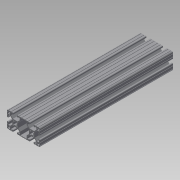
# Autodesk Inventor part: 1530-UL
Saved by Autodesk Inventor 2013 (Build 170138000, 138)
## iProperties
Company: 80/20 Inc.
Created: 2014-04-23
Part Number: 1530-UL
Material: Generic
Document SubType Name: Modeling
Density: 1 g/cm^3
Vendor: 80/20 Inc.
Engineer: Ross Bowman
Designer: Ross Bowman
Catalog Web Link: 8020.net
Material: 6105-T5 Aluminum
Author: Ross Bowman
Keywords: 80/20 , 8020 , T-Slot , Extrusion
Autodesk Inventor part; units mm, degrees
ref_plane "YZ Plane" through (0, 0, 0) normal (1, 0, 0) x (0, 1, 0)
ref_plane "XZ Plane" through (0, 0, 0) normal (0, 1, 0) x (-1, 0, 0)
ref_plane "XY Plane" through (0, 0, 0) normal (0, 0, 1) x (1, 0, 0)
sketch "Sketch1" plane through (0, 0, 0) normal (0, 0, 1) x (1, 0, 0)
  arc A0 (17.2466, -12.2428) -> (16.8656, -11.8618) centre (16.8656, -12.2428) ccw
  line L0 (17.2466, -14.4526) -> (17.2466, -12.2428)
  arc A1 (14.4526, -17.2466) -> (17.2466, -14.4526) centre (14.4526, -14.4526) ccw
  line L1 (12.2428, -17.2466) -> (14.4526, -17.2466)
  arc A2 (11.8618, -16.8656) -> (12.2428, -17.2466) centre (12.2428, -16.8656) ccw
  line L2 (11.8618, -15.0876) -> (11.8618, -16.8656)
  line L3 (12.3952, -14.5542) -> (11.8618, -15.0876)
  line L4 (11.8618, -14.0208) -> (12.3952, -14.5542)
  line L5 (11.8618, -12.2428) -> (11.8618, -14.0208)
  arc A3 (12.2428, -11.8618) -> (11.8618, -12.2428) centre (12.2428, -12.2428) ccw
  line L6 (14.0208, -11.8618) -> (12.2428, -11.8618)
  line L7 (14.5542, -12.3952) -> (14.0208, -11.8618)
  line L8 (15.0876, -11.8618) -> (14.5542, -12.3952)
  line L9 (16.8656, -11.8618) -> (15.0876, -11.8618)
  arc A4 (-3.1119, 1.178) -> (-3.1119, -1.178) centre (0, 0) ccw
  arc A5 (-3.1119, 1.178) -> (-3.1988, 1.5823) centre (-3.4682, 1.3129) ccw
  line L10 (-4.9085, 3.2921) -> (-3.1988, 1.5823)
  arc A6 (-5.1689, 3.9207) -> (-4.9085, 3.2921) centre (-4.2799, 3.9207) ccw
  line L11 (-5.1689, 4.9149) -> (-5.1689, 3.9207)
  arc A7 (-4.9149, 5.1689) -> (-5.1689, 4.9149) centre (-4.9149, 4.9149) ccw
  line L12 (-3.9207, 5.1689) -> (-4.9149, 5.1689)
  arc A8 (-3.2921, 4.9085) -> (-3.9207, 5.1689) centre (-3.9207, 4.2799) ccw
  line L13 (-1.5823, 3.1988) -> (-3.2921, 4.9085)
  arc A9 (-1.5823, 3.1988) -> (-1.178, 3.1119) centre (-1.3129, 3.4682) ccw
  arc A10 (1.178, 3.1119) -> (-1.178, 3.1119) centre (0, 0) ccw
  arc A11 (1.178, 3.1119) -> (1.5823, 3.1988) centre (1.3129, 3.4682) ccw
  line L14 (3.2921, 4.9085) -> (1.5823, 3.1988)
  arc A12 (3.9207, 5.1689) -> (3.2921, 4.9085) centre (3.9207, 4.2799) ccw
  line L15 (4.9149, 5.1689) -> (3.9207, 5.1689)
  arc A13 (5.1689, 4.9149) -> (4.9149, 5.1689) centre (4.9149, 4.9149) ccw
  line L16 (5.1689, 3.9207) -> (5.1689, 4.9149)
  arc A14 (4.9085, 3.2921) -> (5.1689, 3.9207) centre (4.2799, 3.9207) ccw
  line L17 (3.1988, 1.5823) -> (4.9085, 3.2921)
  arc A15 (3.1988, 1.5823) -> (3.1119, 1.178) centre (3.4682, 1.3129) ccw
  arc A16 (3.1119, -1.178) -> (3.1119, 1.178) centre (0, 0) ccw
  arc A17 (3.1119, -1.178) -> (3.1988, -1.5823) centre (3.4682, -1.3129) ccw
  line L18 (4.9085, -3.2921) -> (3.1988, -1.5823)
  arc A18 (5.1689, -3.9207) -> (4.9085, -3.2921) centre (4.2799, -3.9207) ccw
  line L19 (5.1689, -4.9149) -> (5.1689, -3.9207)
  arc A19 (4.9149, -5.1689) -> (5.1689, -4.9149) centre (4.9149, -4.9149) ccw
  line L20 (3.9207, -5.1689) -> (4.9149, -5.1689)
  arc A20 (3.2921, -4.9085) -> (3.9207, -5.1689) centre (3.9207, -4.2799) ccw
  line L21 (1.5823, -3.1988) -> (3.2921, -4.9085)
  arc A21 (1.5823, -3.1988) -> (1.178, -3.1119) centre (1.3129, -3.4682) ccw
  arc A22 (-1.178, -3.1119) -> (1.178, -3.1119) centre (0, 0) ccw
  arc A23 (-1.178, -3.1119) -> (-1.5823, -3.1988) centre (-1.3129, -3.4682) ccw
  line L22 (-3.2921, -4.9085) -> (-1.5823, -3.1988)
  arc A24 (-3.9207, -5.1689) -> (-3.2921, -4.9085) centre (-3.9207, -4.2799) ccw
  line L23 (-4.9149, -5.1689) -> (-3.9207, -5.1689)
  arc A25 (-5.1689, -4.9149) -> (-4.9149, -5.1689) centre (-4.9149, -4.9149) ccw
  line L24 (-5.1689, -3.9207) -> (-5.1689, -4.9149)
  arc A26 (-4.9085, -3.2921) -> (-5.1689, -3.9207) centre (-4.2799, -3.9207) ccw
  line L25 (-3.1988, -1.5823) -> (-4.9085, -3.2921)
  arc A27 (-3.1988, -1.5823) -> (-3.1119, -1.178) centre (-3.4682, -1.3129) ccw
  arc A28 (-41.2119, 1.178) -> (-41.2119, -1.178) centre (-38.1, 0) ccw
  arc A29 (-41.2119, 1.178) -> (-41.2988, 1.5823) centre (-41.5682, 1.3129) ccw
  line L26 (-43.0085, 3.2921) -> (-41.2988, 1.5823)
  arc A30 (-43.2689, 3.9207) -> (-43.0085, 3.2921) centre (-42.3799, 3.9207) ccw
  line L27 (-43.2689, 4.9149) -> (-43.2689, 3.9207)
  arc A31 (-43.0149, 5.1689) -> (-43.2689, 4.9149) centre (-43.0149, 4.9149) ccw
  line L28 (-42.0207, 5.1689) -> (-43.0149, 5.1689)
  arc A32 (-41.3921, 4.9085) -> (-42.0207, 5.1689) centre (-42.0207, 4.2799) ccw
  line L29 (-39.6823, 3.1988) -> (-41.3921, 4.9085)
  arc A33 (-39.6823, 3.1988) -> (-39.278, 3.1119) centre (-39.4129, 3.4682) ccw
  arc A34 (-36.922, 3.1119) -> (-39.278, 3.1119) centre (-38.1, 0) ccw
  arc A35 (-36.922, 3.1119) -> (-36.5177, 3.1988) centre (-36.7871, 3.4682) ccw
  line L30 (-34.8079, 4.9085) -> (-36.5177, 3.1988)
  arc A36 (-34.1793, 5.1689) -> (-34.8079, 4.9085) centre (-34.1793, 4.2799) ccw
  line L31 (-33.1851, 5.1689) -> (-34.1793, 5.1689)
  arc A37 (-32.9311, 4.9149) -> (-33.1851, 5.1689) centre (-33.1851, 4.9149) ccw
  line L32 (-32.9311, 3.9207) -> (-32.9311, 4.9149)
  arc A38 (-33.1915, 3.2921) -> (-32.9311, 3.9207) centre (-33.8201, 3.9207) ccw
  line L33 (-34.9012, 1.5823) -> (-33.1915, 3.2921)
  arc A39 (-34.9012, 1.5823) -> (-34.9881, 1.178) centre (-34.6318, 1.3129) ccw
  arc A40 (-34.9881, -1.178) -> (-34.9881, 1.178) centre (-38.1, 0) ccw
  arc A41 (-34.9881, -1.178) -> (-34.9012, -1.5823) centre (-34.6318, -1.3129) ccw
  line L34 (-33.1915, -3.2921) -> (-34.9012, -1.5823)
  arc A42 (-32.9311, -3.9207) -> (-33.1915, -3.2921) centre (-33.8201, -3.9207) ccw
  line L35 (-32.9311, -4.9149) -> (-32.9311, -3.9207)
  arc A43 (-33.1851, -5.1689) -> (-32.9311, -4.9149) centre (-33.1851, -4.9149) ccw
  line L36 (-34.1793, -5.1689) -> (-33.1851, -5.1689)
  arc A44 (-34.8079, -4.9085) -> (-34.1793, -5.1689) centre (-34.1793, -4.2799) ccw
  line L37 (-36.5177, -3.1988) -> (-34.8079, -4.9085)
  arc A45 (-36.5177, -3.1988) -> (-36.922, -3.1119) centre (-36.7871, -3.4682) ccw
  arc A46 (-39.278, -3.1119) -> (-36.922, -3.1119) centre (-38.1, 0) ccw
  arc A47 (-39.278, -3.1119) -> (-39.6823, -3.1988) centre (-39.4129, -3.4682) ccw
  line L38 (-41.3921, -4.9085) -> (-39.6823, -3.1988)
  arc A48 (-42.0207, -5.1689) -> (-41.3921, -4.9085) centre (-42.0207, -4.2799) ccw
  line L39 (-43.0149, -5.1689) -> (-42.0207, -5.1689)
  arc A49 (-43.2689, -4.9149) -> (-43.0149, -5.1689) centre (-43.0149, -4.9149) ccw
  line L40 (-43.2689, -3.9207) -> (-43.2689, -4.9149)
  arc A50 (-43.0085, -3.2921) -> (-43.2689, -3.9207) centre (-42.3799, -3.9207) ccw
  line L41 (-41.2988, -1.5823) -> (-43.0085, -3.2921)
  arc A51 (-41.2988, -1.5823) -> (-41.2119, -1.178) centre (-41.5682, -1.3129) ccw
  arc A52 (-54.9656, -11.8618) -> (-55.3466, -12.2428) centre (-54.9656, -12.2428) ccw
  line L42 (-53.1876, -11.8618) -> (-54.9656, -11.8618)
  line L43 (-52.6542, -12.3952) -> (-53.1876, -11.8618)
  line L44 (-52.1208, -11.8618) -> (-52.6542, -12.3952)
  line L45 (-50.3428, -11.8618) -> (-52.1208, -11.8618)
  arc A53 (-49.9618, -12.2428) -> (-50.3428, -11.8618) centre (-50.3428, -12.2428) ccw
  line L46 (-49.9618, -14.0208) -> (-49.9618, -12.2428)
  line L47 (-50.4952, -14.5542) -> (-49.9618, -14.0208)
  line L48 (-49.9618, -15.0876) -> (-50.4952, -14.5542)
  line L49 (-49.9618, -16.8656) -> (-49.9618, -15.0876)
  arc A54 (-50.3428, -17.2466) -> (-49.9618, -16.8656) centre (-50.3428, -16.8656) ccw
  line L50 (-52.5526, -17.2466) -> (-50.3428, -17.2466)
  arc A55 (-55.3466, -14.4526) -> (-52.5526, -17.2466) centre (-52.5526, -14.4526) ccw
  line L51 (-55.3466, -12.2428) -> (-55.3466, -14.4526)
  arc A56 (-55.3466, 12.2428) -> (-54.9656, 11.8618) centre (-54.9656, 12.2428) ccw
  line L52 (-55.3466, 14.4526) -> (-55.3466, 12.2428)
  arc A57 (-52.5526, 17.2466) -> (-55.3466, 14.4526) centre (-52.5526, 14.4526) ccw
  line L53 (-50.3428, 17.2466) -> (-52.5526, 17.2466)
  arc A58 (-49.9618, 16.8656) -> (-50.3428, 17.2466) centre (-50.3428, 16.8656) ccw
  line L54 (-49.9618, 15.0876) -> (-49.9618, 16.8656)
  line L55 (-50.4952, 14.5542) -> (-49.9618, 15.0876)
  line L56 (-49.9618, 14.0208) -> (-50.4952, 14.5542)
  line L57 (-49.9618, 12.2428) -> (-49.9618, 14.0208)
  arc A59 (-50.3428, 11.8618) -> (-49.9618, 12.2428) centre (-50.3428, 12.2428) ccw
  line L58 (-52.1208, 11.8618) -> (-50.3428, 11.8618)
  line L59 (-52.6542, 12.3952) -> (-52.1208, 11.8618)
  line L60 (-53.1876, 11.8618) -> (-52.6542, 12.3952)
  line L61 (-54.9656, 11.8618) -> (-53.1876, 11.8618)
  arc A60 (-25.8572, 17.2466) -> (-26.2382, 16.8656) centre (-25.8572, 16.8656) ccw
  line L62 (-12.2428, 17.2466) -> (-25.8572, 17.2466)
  arc A61 (-11.8618, 16.8656) -> (-12.2428, 17.2466) centre (-12.2428, 16.8656) ccw
  line L63 (-11.8618, 10.8253) -> (-11.8618, 16.8656)
  arc A62 (-11.8618, 10.8253) -> (-11.4898, 9.9273) centre (-10.5918, 10.8253) ccw
  line L64 (-7.1157, 5.5531) -> (-11.4898, 9.9273)
  arc A63 (-6.7437, 4.6551) -> (-7.1157, 5.5531) centre (-8.0137, 4.6551) ccw
  line L65 (-6.7437, -4.6551) -> (-6.7437, 4.6551)
  arc A64 (-7.1157, -5.5531) -> (-6.7437, -4.6551) centre (-8.0137, -4.6551) ccw
  line L66 (-11.4898, -9.9273) -> (-7.1157, -5.5531)
  arc A65 (-11.4898, -9.9273) -> (-11.8618, -10.8253) centre (-10.5918, -10.8253) ccw
  line L67 (-11.8618, -16.8656) -> (-11.8618, -10.8253)
  arc A66 (-12.2428, -17.2466) -> (-11.8618, -16.8656) centre (-12.2428, -16.8656) ccw
  line L68 (-25.8572, -17.2466) -> (-12.2428, -17.2466)
  arc A67 (-26.2382, -16.8656) -> (-25.8572, -17.2466) centre (-25.8572, -16.8656) ccw
  line L69 (-26.2382, -10.8253) -> (-26.2382, -16.8656)
  arc A68 (-26.2382, -10.8253) -> (-26.6102, -9.9273) centre (-27.5082, -10.8253) ccw
  line L70 (-30.9843, -5.5531) -> (-26.6102, -9.9273)
  arc A69 (-31.3563, -4.6551) -> (-30.9843, -5.5531) centre (-30.0863, -4.6551) ccw
  line L71 (-31.3563, 4.6551) -> (-31.3563, -4.6551)
  arc A70 (-30.9843, 5.5531) -> (-31.3563, 4.6551) centre (-30.0863, 4.6551) ccw
  line L72 (-26.6102, 9.9273) -> (-30.9843, 5.5531)
  arc A71 (-26.6102, 9.9273) -> (-26.2382, 10.8253) centre (-27.5082, 10.8253) ccw
  line L73 (-26.2382, 16.8656) -> (-26.2382, 10.8253)
  arc A72 (16.8656, 11.8618) -> (17.2466, 12.2428) centre (16.8656, 12.2428) ccw
  line L74 (15.0876, 11.8618) -> (16.8656, 11.8618)
  line L75 (14.5542, 12.3952) -> (15.0876, 11.8618)
  line L76 (14.0208, 11.8618) -> (14.5542, 12.3952)
  line L77 (12.2428, 11.8618) -> (14.0208, 11.8618)
  arc A73 (11.8618, 12.2428) -> (12.2428, 11.8618) centre (12.2428, 12.2428) ccw
  line L78 (11.8618, 14.0208) -> (11.8618, 12.2428)
  line L79 (12.3952, 14.5542) -> (11.8618, 14.0208)
  line L80 (11.8618, 15.0876) -> (12.3952, 14.5542)
  line L81 (11.8618, 16.8656) -> (11.8618, 15.0876)
  arc A74 (12.2428, 17.2466) -> (11.8618, 16.8656) centre (12.2428, 16.8656) ccw
  line L82 (14.4526, 17.2466) -> (12.2428, 17.2466)
  arc A75 (17.2466, 14.4526) -> (14.4526, 17.2466) centre (14.4526, 14.4526) ccw
  line L83 (17.2466, 12.2428) -> (17.2466, 14.4526)
  arc A76 (-15.8496, 19.05) -> (-14.3256, 19.05) centre (-15.0876, 19.05) ccw
  line L84 (-15.8496, 19.05) -> (-22.2504, 19.05)
  arc A77 (-23.7744, 19.05) -> (-22.2504, 19.05) centre (-23.0124, 19.05) ccw
  line L85 (-23.7744, 19.05) -> (-28.6004, 19.05)
  arc A78 (-30.1244, 19.05) -> (-28.6004, 19.05) centre (-29.3624, 19.05) ccw
  line L86 (-30.1244, 19.05) -> (-32.4612, 19.05)
  arc A79 (-32.4612, 19.05) -> (-34.036, 17.4752) centre (-32.4612, 17.4752) ccw
  line L87 (-34.036, 17.4752) -> (-34.036, 16.5608)
  arc A80 (-34.036, 16.5608) -> (-32.4612, 14.986) centre (-32.4612, 16.5608) ccw
  line L88 (-32.4612, 14.986) -> (-31.623, 14.986)
  arc A81 (-31.623, 14.986) -> (-31.242, 15.367) centre (-31.623, 15.367) ccw
  line L89 (-31.242, 15.367) -> (-31.242, 15.6972)
  arc A82 (-30.861, 16.0782) -> (-31.242, 15.6972) centre (-30.861, 15.6972) ccw
  line L90 (-30.861, 16.0782) -> (-28.702, 16.0782)
  arc A83 (-27.813, 15.1892) -> (-28.702, 16.0782) centre (-28.702, 15.1892) ccw
  line L91 (-27.813, 15.1892) -> (-27.813, 12.3756)
  arc A84 (-28.185, 11.4776) -> (-27.813, 12.3756) centre (-29.083, 12.3756) ccw
  line L92 (-28.185, 11.4776) -> (-32.5469, 7.1157)
  arc A85 (-33.4449, 6.7437) -> (-32.5469, 7.1157) centre (-33.4449, 8.0137) ccw
  line L93 (-33.4449, 6.7437) -> (-42.7551, 6.7437)
  arc A86 (-43.6531, 7.1157) -> (-42.7551, 6.7437) centre (-42.7551, 8.0137) ccw
  line L94 (-43.6531, 7.1157) -> (-48.015, 11.4776)
  arc A87 (-48.387, 12.3756) -> (-48.015, 11.4776) centre (-47.117, 12.3756) ccw
  line L95 (-48.387, 12.3756) -> (-48.387, 15.1892)
  arc A88 (-47.498, 16.0782) -> (-48.387, 15.1892) centre (-47.498, 15.1892) ccw
  line L96 (-47.498, 16.0782) -> (-45.339, 16.0782)
  arc A89 (-44.958, 15.6972) -> (-45.339, 16.0782) centre (-45.339, 15.6972) ccw
  line L97 (-44.958, 15.6972) -> (-44.958, 15.367)
  arc A90 (-44.958, 15.367) -> (-44.577, 14.986) centre (-44.577, 15.367) ccw
  line L98 (-44.577, 14.986) -> (-43.7388, 14.986)
  arc A91 (-43.7388, 14.986) -> (-42.164, 16.5608) centre (-43.7388, 16.5608) ccw
  line L99 (-42.164, 16.5608) -> (-42.164, 17.4752)
  arc A92 (-42.164, 17.4752) -> (-43.7388, 19.05) centre (-43.7388, 17.4752) ccw
  line L100 (-43.7388, 19.05) -> (-46.0756, 19.05)
  arc A93 (-47.5996, 19.05) -> (-46.0756, 19.05) centre (-46.8376, 19.05) ccw
  line L101 (-47.5996, 19.05) -> (-52.4256, 19.05)
  arc A94 (-53.9496, 19.05) -> (-52.4256, 19.05) centre (-53.1876, 19.05) ccw
  line L102 (-53.9496, 19.05) -> (-53.975, 19.05)
  arc A95 (-53.975, 19.05) -> (-57.15, 15.875) centre (-53.975, 15.875) ccw
  line L103 (-57.15, 15.875) -> (-57.15, 15.8496)
  arc A96 (-57.15, 14.3256) -> (-57.15, 15.8496) centre (-57.15, 15.0876) ccw
  line L104 (-57.15, 14.3256) -> (-57.15, 9.4996)
  arc A97 (-57.15, 7.9756) -> (-57.15, 9.4996) centre (-57.15, 8.7376) ccw
  line L105 (-57.15, 7.9756) -> (-57.15, 5.6388)
  arc A98 (-57.15, 5.6388) -> (-55.5752, 4.064) centre (-55.5752, 5.6388) ccw
  line L106 (-55.5752, 4.064) -> (-54.6608, 4.064)
  arc A99 (-54.6608, 4.064) -> (-53.086, 5.6388) centre (-54.6608, 5.6388) ccw
  line L107 (-53.086, 5.6388) -> (-53.086, 6.477)
  arc A100 (-53.086, 6.477) -> (-53.467, 6.858) centre (-53.467, 6.477) ccw
  line L108 (-53.467, 6.858) -> (-53.7972, 6.858)
  arc A101 (-54.1782, 7.239) -> (-53.7972, 6.858) centre (-53.7972, 7.239) ccw
  line L109 (-54.1782, 7.239) -> (-54.1782, 9.398)
  arc A102 (-53.2892, 10.287) -> (-54.1782, 9.398) centre (-53.2892, 9.398) ccw
  line L110 (-53.2892, 10.287) -> (-50.4756, 10.287)
  arc A103 (-49.5776, 9.915) -> (-50.4756, 10.287) centre (-50.4756, 9.017) ccw
  line L111 (-49.5776, 9.915) -> (-45.2157, 5.5531)
  arc A104 (-44.8437, 4.6551) -> (-45.2157, 5.5531) centre (-46.1137, 4.6551) ccw
  line L112 (-44.8437, 4.6551) -> (-44.8437, -4.6551)
  arc A105 (-45.2157, -5.5531) -> (-44.8437, -4.6551) centre (-46.1137, -4.6551) ccw
  line L113 (-45.2157, -5.5531) -> (-49.5776, -9.915)
  arc A106 (-50.4756, -10.287) -> (-49.5776, -9.915) centre (-50.4756, -9.017) ccw
  line L114 (-50.4756, -10.287) -> (-53.2892, -10.287)
  arc A107 (-54.1782, -9.398) -> (-53.2892, -10.287) centre (-53.2892, -9.398) ccw
  line L115 (-54.1782, -9.398) -> (-54.1782, -7.239)
  arc A108 (-53.7972, -6.858) -> (-54.1782, -7.239) centre (-53.7972, -7.239) ccw
  line L116 (-53.7972, -6.858) -> (-53.467, -6.858)
  arc A109 (-53.467, -6.858) -> (-53.086, -6.477) centre (-53.467, -6.477) ccw
  line L117 (-53.086, -6.477) -> (-53.086, -5.6388)
  arc A110 (-53.086, -5.6388) -> (-54.6608, -4.064) centre (-54.6608, -5.6388) ccw
  line L118 (-54.6608, -4.064) -> (-55.5752, -4.064)
  arc A111 (-55.5752, -4.064) -> (-57.15, -5.6388) centre (-55.5752, -5.6388) ccw
  line L119 (-57.15, -5.6388) -> (-57.15, -7.9756)
  arc A112 (-57.15, -9.4996) -> (-57.15, -7.9756) centre (-57.15, -8.7376) ccw
  line L120 (-57.15, -9.4996) -> (-57.15, -14.3256)
  arc A113 (-57.15, -15.8496) -> (-57.15, -14.3256) centre (-57.15, -15.0876) ccw
  line L121 (-57.15, -15.8496) -> (-57.15, -15.875)
  arc A114 (-57.15, -15.875) -> (-53.975, -19.05) centre (-53.975, -15.875) ccw
  line L122 (-53.975, -19.05) -> (-53.9496, -19.05)
  arc A115 (-52.4256, -19.05) -> (-53.9496, -19.05) centre (-53.1876, -19.05) ccw
  line L123 (-52.4256, -19.05) -> (-47.5996, -19.05)
  arc A116 (-46.0756, -19.05) -> (-47.5996, -19.05) centre (-46.8376, -19.05) ccw
  line L124 (-46.0756, -19.05) -> (-43.7388, -19.05)
  arc A117 (-43.7388, -19.05) -> (-42.164, -17.4752) centre (-43.7388, -17.4752) ccw
  line L125 (-42.164, -17.4752) -> (-42.164, -16.5608)
  arc A118 (-42.164, -16.5608) -> (-43.7388, -14.986) centre (-43.7388, -16.5608) ccw
  line L126 (-43.7388, -14.986) -> (-44.577, -14.986)
  arc A119 (-44.577, -14.986) -> (-44.958, -15.367) centre (-44.577, -15.367) ccw
  line L127 (-44.958, -15.367) -> (-44.958, -15.6972)
  arc A120 (-45.339, -16.0782) -> (-44.958, -15.6972) centre (-45.339, -15.6972) ccw
  line L128 (-45.339, -16.0782) -> (-47.498, -16.0782)
  arc A121 (-48.387, -15.1892) -> (-47.498, -16.0782) centre (-47.498, -15.1892) ccw
  line L129 (-48.387, -15.1892) -> (-48.387, -12.3756)
  arc A122 (-48.015, -11.4776) -> (-48.387, -12.3756) centre (-47.117, -12.3756) ccw
  line L130 (-48.015, -11.4776) -> (-43.6531, -7.1157)
  arc A123 (-42.7551, -6.7437) -> (-43.6531, -7.1157) centre (-42.7551, -8.0137) ccw
  line L131 (-42.7551, -6.7437) -> (-33.4449, -6.7437)
  arc A124 (-32.5469, -7.1157) -> (-33.4449, -6.7437) centre (-33.4449, -8.0137) ccw
  line L132 (-32.5469, -7.1157) -> (-28.185, -11.4776)
  arc A125 (-27.813, -12.3756) -> (-28.185, -11.4776) centre (-29.083, -12.3756) ccw
  line L133 (-27.813, -12.3756) -> (-27.813, -15.1892)
  arc A126 (-28.702, -16.0782) -> (-27.813, -15.1892) centre (-28.702, -15.1892) ccw
  line L134 (-28.702, -16.0782) -> (-30.861, -16.0782)
  arc A127 (-31.242, -15.6972) -> (-30.861, -16.0782) centre (-30.861, -15.6972) ccw
  line L135 (-31.242, -15.6972) -> (-31.242, -15.367)
  arc A128 (-31.242, -15.367) -> (-31.623, -14.986) centre (-31.623, -15.367) ccw
  line L136 (-31.623, -14.986) -> (-32.4612, -14.986)
  arc A129 (-32.4612, -14.986) -> (-34.036, -16.5608) centre (-32.4612, -16.5608) ccw
  line L137 (-34.036, -16.5608) -> (-34.036, -17.4752)
  arc A130 (-34.036, -17.4752) -> (-32.4612, -19.05) centre (-32.4612, -17.4752) ccw
  line L138 (-32.4612, -19.05) -> (-30.1244, -19.05)
  arc A131 (-28.6004, -19.05) -> (-30.1244, -19.05) centre (-29.3624, -19.05) ccw
  line L139 (-28.6004, -19.05) -> (-23.7744, -19.05)
  arc A132 (-22.2504, -19.05) -> (-23.7744, -19.05) centre (-23.0124, -19.05) ccw
  line L140 (-22.2504, -19.05) -> (-15.8496, -19.05)
  arc A133 (-14.3256, -19.05) -> (-15.8496, -19.05) centre (-15.0876, -19.05) ccw
  line L141 (-14.3256, -19.05) -> (-9.4996, -19.05)
  arc A134 (-7.9756, -19.05) -> (-9.4996, -19.05) centre (-8.7376, -19.05) ccw
  line L142 (-7.9756, -19.05) -> (-5.6388, -19.05)
  arc A135 (-5.6388, -19.05) -> (-4.064, -17.4752) centre (-5.6388, -17.4752) ccw
  line L143 (-4.064, -17.4752) -> (-4.064, -16.5608)
  arc A136 (-4.064, -16.5608) -> (-5.6388, -14.986) centre (-5.6388, -16.5608) ccw
  line L144 (-5.6388, -14.986) -> (-6.477, -14.986)
  arc A137 (-6.477, -14.986) -> (-6.858, -15.367) centre (-6.477, -15.367) ccw
  line L145 (-6.858, -15.367) -> (-6.858, -15.6972)
  arc A138 (-7.239, -16.0782) -> (-6.858, -15.6972) centre (-7.239, -15.6972) ccw
  line L146 (-7.239, -16.0782) -> (-9.398, -16.0782)
  arc A139 (-10.287, -15.1892) -> (-9.398, -16.0782) centre (-9.398, -15.1892) ccw
  line L147 (-10.287, -15.1892) -> (-10.287, -12.3756)
  arc A140 (-9.915, -11.4776) -> (-10.287, -12.3756) centre (-9.017, -12.3756) ccw
  line L148 (-9.915, -11.4776) -> (-5.5531, -7.1157)
  arc A141 (-4.6551, -6.7437) -> (-5.5531, -7.1157) centre (-4.6551, -8.0137) ccw
  line L149 (-4.6551, -6.7437) -> (4.6551, -6.7437)
  arc A142 (5.5531, -7.1157) -> (4.6551, -6.7437) centre (4.6551, -8.0137) ccw
  line L150 (5.5531, -7.1157) -> (9.915, -11.4776)
  arc A143 (10.287, -12.3756) -> (9.915, -11.4776) centre (9.017, -12.3756) ccw
  line L151 (10.287, -12.3756) -> (10.287, -15.1892)
  arc A144 (9.398, -16.0782) -> (10.287, -15.1892) centre (9.398, -15.1892) ccw
  line L152 (9.398, -16.0782) -> (7.239, -16.0782)
  arc A145 (6.858, -15.6972) -> (7.239, -16.0782) centre (7.239, -15.6972) ccw
  line L153 (6.858, -15.6972) -> (6.858, -15.367)
  arc A146 (6.858, -15.367) -> (6.477, -14.986) centre (6.477, -15.367) ccw
  line L154 (6.477, -14.986) -> (5.6388, -14.986)
  arc A147 (5.6388, -14.986) -> (4.064, -16.5608) centre (5.6388, -16.5608) ccw
  line L155 (4.064, -16.5608) -> (4.064, -17.4752)
  arc A148 (4.064, -17.4752) -> (5.6388, -19.05) centre (5.6388, -17.4752) ccw
  line L156 (5.6388, -19.05) -> (7.9756, -19.05)
  arc A149 (9.4996, -19.05) -> (7.9756, -19.05) centre (8.7376, -19.05) ccw
  line L157 (9.4996, -19.05) -> (14.3256, -19.05)
  arc A150 (15.8496, -19.05) -> (14.3256, -19.05) centre (15.0876, -19.05) ccw
  line L158 (15.8496, -19.05) -> (15.875, -19.05)
  arc A151 (15.875, -19.05) -> (19.05, -15.875) centre (15.875, -15.875) ccw
  line L159 (19.05, -15.875) -> (19.05, -15.8496)
  arc A152 (19.05, -14.3256) -> (19.05, -15.8496) centre (19.05, -15.0876) ccw
  line L160 (19.05, -14.3256) -> (19.05, -9.4996)
  arc A153 (19.05, -7.9756) -> (19.05, -9.4996) centre (19.05, -8.7376) ccw
  line L161 (19.05, -7.9756) -> (19.05, -5.6388)
  arc A154 (19.05, -5.6388) -> (17.4752, -4.064) centre (17.4752, -5.6388) ccw
  line L162 (17.4752, -4.064) -> (16.5608, -4.064)
  arc A155 (16.5608, -4.064) -> (14.986, -5.6388) centre (16.5608, -5.6388) ccw
  line L163 (14.986, -5.6388) -> (14.986, -6.477)
  arc A156 (14.986, -6.477) -> (15.367, -6.858) centre (15.367, -6.477) ccw
  line L164 (15.367, -6.858) -> (15.6972, -6.858)
  arc A157 (16.0782, -7.239) -> (15.6972, -6.858) centre (15.6972, -7.239) ccw
  line L165 (16.0782, -7.239) -> (16.0782, -9.398)
  arc A158 (15.1892, -10.287) -> (16.0782, -9.398) centre (15.1892, -9.398) ccw
  line L166 (15.1892, -10.287) -> (12.3756, -10.287)
  arc A159 (11.4776, -9.915) -> (12.3756, -10.287) centre (12.3756, -9.017) ccw
  line L167 (11.4776, -9.915) -> (7.1157, -5.5531)
  arc A160 (6.7437, -4.6551) -> (7.1157, -5.5531) centre (8.0137, -4.6551) ccw
  line L168 (6.7437, -4.6551) -> (6.7437, 4.6551)
  arc A161 (7.1157, 5.5531) -> (6.7437, 4.6551) centre (8.0137, 4.6551) ccw
  line L169 (7.1157, 5.5531) -> (11.4776, 9.915)
  arc A162 (12.3756, 10.287) -> (11.4776, 9.915) centre (12.3756, 9.017) ccw
  line L170 (12.3756, 10.287) -> (15.1892, 10.287)
  arc A163 (16.0782, 9.398) -> (15.1892, 10.287) centre (15.1892, 9.398) ccw
  line L171 (16.0782, 9.398) -> (16.0782, 7.239)
  arc A164 (15.6972, 6.858) -> (16.0782, 7.239) centre (15.6972, 7.239) ccw
  line L172 (15.6972, 6.858) -> (15.367, 6.858)
  arc A165 (15.367, 6.858) -> (14.986, 6.477) centre (15.367, 6.477) ccw
  line L173 (14.986, 6.477) -> (14.986, 5.6388)
  arc A166 (14.986, 5.6388) -> (16.5608, 4.064) centre (16.5608, 5.6388) ccw
  line L174 (16.5608, 4.064) -> (17.4752, 4.064)
  arc A167 (17.4752, 4.064) -> (19.05, 5.6388) centre (17.4752, 5.6388) ccw
  line L175 (19.05, 5.6388) -> (19.05, 7.9756)
  arc A168 (19.05, 9.4996) -> (19.05, 7.9756) centre (19.05, 8.7376) ccw
  line L176 (19.05, 9.4996) -> (19.05, 14.3256)
  arc A169 (19.05, 15.8496) -> (19.05, 14.3256) centre (19.05, 15.0876) ccw
  line L177 (19.05, 15.8496) -> (19.05, 15.875)
  arc A170 (19.05, 15.875) -> (15.875, 19.05) centre (15.875, 15.875) ccw
  line L178 (15.875, 19.05) -> (15.8496, 19.05)
  arc A171 (14.3256, 19.05) -> (15.8496, 19.05) centre (15.0876, 19.05) ccw
  line L179 (14.3256, 19.05) -> (9.4996, 19.05)
  arc A172 (7.9756, 19.05) -> (9.4996, 19.05) centre (8.7376, 19.05) ccw
  line L180 (7.9756, 19.05) -> (5.6388, 19.05)
  arc A173 (5.6388, 19.05) -> (4.064, 17.4752) centre (5.6388, 17.4752) ccw
  line L181 (4.064, 17.4752) -> (4.064, 16.5608)
  arc A174 (4.064, 16.5608) -> (5.6388, 14.986) centre (5.6388, 16.5608) ccw
  line L182 (5.6388, 14.986) -> (6.477, 14.986)
  arc A175 (6.477, 14.986) -> (6.858, 15.367) centre (6.477, 15.367) ccw
  line L183 (6.858, 15.367) -> (6.858, 15.6972)
  arc A176 (7.239, 16.0782) -> (6.858, 15.6972) centre (7.239, 15.6972) ccw
  line L184 (7.239, 16.0782) -> (9.398, 16.0782)
  arc A177 (10.287, 15.1892) -> (9.398, 16.0782) centre (9.398, 15.1892) ccw
  line L185 (10.287, 15.1892) -> (10.287, 12.3756)
  arc A178 (9.915, 11.4776) -> (10.287, 12.3756) centre (9.017, 12.3756) ccw
  line L186 (9.915, 11.4776) -> (5.5531, 7.1157)
  arc A179 (4.6551, 6.7437) -> (5.5531, 7.1157) centre (4.6551, 8.0137) ccw
  line L187 (4.6551, 6.7437) -> (-4.6551, 6.7437)
  arc A180 (-5.5531, 7.1157) -> (-4.6551, 6.7437) centre (-4.6551, 8.0137) ccw
  line L188 (-5.5531, 7.1157) -> (-9.915, 11.4776)
  arc A181 (-10.287, 12.3756) -> (-9.915, 11.4776) centre (-9.017, 12.3756) ccw
  line L189 (-10.287, 12.3756) -> (-10.287, 15.1892)
  arc A182 (-9.398, 16.0782) -> (-10.287, 15.1892) centre (-9.398, 15.1892) ccw
  line L190 (-9.398, 16.0782) -> (-7.239, 16.0782)
  arc A183 (-6.858, 15.6972) -> (-7.239, 16.0782) centre (-7.239, 15.6972) ccw
  line L191 (-6.858, 15.6972) -> (-6.858, 15.367)
  arc A184 (-6.858, 15.367) -> (-6.477, 14.986) centre (-6.477, 15.367) ccw
  line L192 (-6.477, 14.986) -> (-5.6388, 14.986)
  arc A185 (-5.6388, 14.986) -> (-4.064, 16.5608) centre (-5.6388, 16.5608) ccw
  line L193 (-4.064, 16.5608) -> (-4.064, 17.4752)
  arc A186 (-4.064, 17.4752) -> (-5.6388, 19.05) centre (-5.6388, 17.4752) ccw
  line L194 (-5.6388, 19.05) -> (-7.9756, 19.05)
  arc A187 (-9.4996, 19.05) -> (-7.9756, 19.05) centre (-8.7376, 19.05) ccw
  line L195 (-9.4996, 19.05) -> (-14.3256, 19.05)
  point P0 (0, 0)
  constraints: 513 tangent, 392 end point, 376 point on circle, 188 centre point, 173 equal radius, 81 parallel, 34 perpendicular, 4 collinear, 2 concentric
extrude "Extrusion1" add sketch "Sketch1" against normal blind 304.8
body "Solid1"
